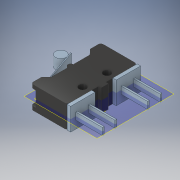
# Autodesk Inventor part: CH_01_0025_end_switch
Saved by Autodesk Inventor 2019 (Build 230136000, 136)
## iProperties
Created: 2022-03-07
Part Number: CH_01_0025_end_switch
Material: Generic
Document SubType Name: Modeling
Designer: Tomasz Krakowski
Density: 1 g/cm^3
Appearance: Default
Author: Tomasz Krakowski
Autodesk Inventor part; units mm, degrees
ref_plane "YZ Plane" through (0, 0, 0) normal (1, 0, 0) x (0, 1, 0)
ref_plane "XZ Plane" through (0, 0, 0) normal (0, 1, 0) x (-1, 0, 0)
ref_plane "XY Plane" through (0, 0, 0) normal (0, 0, 1) x (1, 0, 0)
sketch "Sketch1" plane through (0, 0, 0) normal (0, 1, 0) x (-1, 0, 0)
  line L0 (0, 0) -> (0, 1)
  line L1 (0, 1) -> (0.75, 1)
  line L2 (0.75, 1) -> (0.75, 9.27)
  line L3 (1.5, 10.02) -> (10.4, 10.02)
  line L4 (11.15, 9.27) -> (11.15, 7.02)
  line L5 (11.15, 7.02) -> (9.75, 5.5)
  line L6 (9.75, 5.5) -> (9.75, 0.75)
  arc A0 (10.5, 0) -> (9.75, 0.75) centre (9.75, 0) ccw
  line L7 (9.75, 0) -> (9.75, 0.75) construction
  circle A1 centre (2.85, 3.5) radius 1.05
  line L8 (9.75, 0) -> (9.25, 0) construction
  line L9 (0, 0) -> (9.25, 0) construction
  line L10 (9.75, 7.7) -> (9.75, 5.5) construction
  arc A2 (11.15, 9.27) -> (10.4, 10.02) centre (10.4, 9.27) ccw
  arc A3 (1.5, 10.02) -> (0.75, 9.27) centre (1.5, 9.27) ccw
  line L11 (9.75, 0) -> (10.5, 0) construction
  line L12 (0, 0) -> (0, -1)
  line L13 (0, -1) -> (0.75, -1)
  line L14 (0.75, -1) -> (0.75, -9.27)
  line L15 (1.5, -10.02) -> (10.4, -10.02)
  line L16 (11.15, -9.27) -> (11.15, -7.02)
  line L17 (11.15, -7.02) -> (9.75, -5.5)
  line L18 (9.75, -5.5) -> (9.75, -0.75)
  arc A4 (9.75, -0.75) -> (10.5, 0) centre (9.75, 0) ccw
  line L19 (9.75, 0) -> (9.75, -0.75) construction
  circle A5 centre (2.85, -3.5) radius 1.05
  line L20 (9.75, -7.7) -> (9.75, -5.5) construction
  arc A6 (10.4, -10.02) -> (11.15, -9.27) centre (10.4, -9.27) ccw
  arc A7 (0.75, -9.27) -> (1.5, -10.02) centre (1.5, -9.27) ccw
  point P0 (11.15, 10.02)
  point P1 (11.15, -10.02)
  dimension "d0" = 0.75
  dimension "d1" = 2.1
  dimension "d2" = 3.5
  dimension "d3" = 10.02
  dimension "d4" = 3
  dimension "d5" = 0.75
  dimension "d6" = 2.1
  dimension "d7" = 1
  dimension "d8" = 6.9
  dimension "d9" = 8.3
  dimension "d10" = 4.2
  dimension "d11" = 5.5
  dimension "d12" = 0.75
  constraints: 42 end point, 14 symmetric about line, 12 point on circle, 8 centre point, 4 perpendicular, 4 point on line, 4 tangent, 3 collinear, 2 horizontal, 1 equal radius, 1 parallel, 1 vertical, 4 other
  measures "d0" distance of L6.end L7.start
  measures "d1" distance from line of L2 A1.centre
  measures "d2" vertical distance of L0.start A1.centre
  measures "d3" distance from line of L0.start L3
  measures "d4" distance of point (11.15, 10.02) L4.end
  measures "d5" distance of L0.end L1.end
  measures "d6" diameter of A1
  measures "d7" distance between parallel lines of L9 L1
  measures "d8" distance from line of A1.centre L6
  measures "d9" distance from line of L4 A1.centre
  measures "d10" vertical distance of A1.centre L10.start
  measures "d11" distance from line of L8 L5.end
  measures "d12" radius of A2
extrude "Extrusion1" add sketch "Sketch1" along normal blind 6.4
sketch "Sketch2" plane through (-0.75, 0, 9.27) normal (1, 0, 0) x (0, 0, -1)
  line L0 (-0.75, 0) -> (0, 0) projected
  line L1 (8.52, 6.4) -> (3.77, 6.4) construction
  line L2 (-0.75, 0) -> (6.25, 0)
  line L3 (6.25, 0) -> (6.25, 6.4)
  line L4 (6.25, 6.4) -> (-0.75, 6.4)
  line L5 (-0.75, 6.4) -> (-0.75, 0)
  line L6 (8.27, 6.4) -> (10.27, 6.4) construction
  line L7 (9.27, 6.4) -> (9.27, 0) construction
  line L8 (19.29, 0) -> (18.54, 0)
  line L9 (19.29, 0) -> (12.29, 0)
  line L10 (12.29, 0) -> (12.29, 6.4)
  line L11 (12.29, 6.4) -> (19.29, 6.4)
  line L12 (19.29, 6.4) -> (19.29, 0)
  point P0 (14.77, 6.4)
  dimension "d15" = 7
  constraints: 20 end point, 6 symmetric about line, 2 parallel, 1 horizontal, 1 midpoint, 1 perpendicular, 1 point on line, 1 vertical
  measures "d15" distance between parallel lines of L5 L3
extrude "Extrusion2" add sketch "Sketch2" along normal blind 1 separate body
sketch "Sketch3" plane through (0.25, 0, 9.27) normal (1, 0, 0) x (0, 0, -1)
  line L0 (0.75, 2.2) -> (1.25, 2.2)
  line L1 (1.25, 2.2) -> (1.25, 4.2)
  line L2 (1.25, 4.2) -> (0.75, 4.2)
  line L3 (0.75, 4.2) -> (0.75, 2.2)
  line L4 (0.75, 2.2) -> (1.25, 4.2) construction
  line L5 (1.25, 2.2) -> (0.75, 4.2) construction
  line L6 (4.35, 2.2) -> (4.85, 2.2)
  line L7 (4.85, 2.2) -> (4.85, 4.2)
  line L8 (4.85, 4.2) -> (4.35, 4.2)
  line L9 (4.35, 4.2) -> (4.35, 2.2)
  line L10 (4.35, 2.2) -> (4.85, 4.2) construction
  line L11 (4.85, 2.2) -> (4.35, 4.2) construction
  line L12 (1, 3.2) -> (4.6, 3.2) construction
  line L13 (-0.75, 0) -> (-0.75, 6.4) construction
  line L14 (-0.75, 3.2) -> (1, 3.2) construction
  point P0 (9.27, 0)
  dimension "d18" = 0.5
  dimension "d19" = 2
  dimension "d21" = 3.6
  dimension "d22" = 1.75
  constraints: 28 end point, 5 midpoint, 4 parallel, 3 collinear, 3 horizontal, 2 perpendicular
  measures "d18" distance of L1.end L2.end
  measures "d19" distance between parallel lines of L0 L2
  measures "d21" distance of L12.end L12.start
  measures "d22" distance of L14.start L12.start
extrude "Extrusion3" add sketch "Sketch3" along normal blind 7.6 bodies 2
mirror "Mirror1" about plane through (0, 0, 0) normal (0, 0, 1) of "Extrusion3" bodies 2
sketch "Sketch4" plane through (-1.5, 0, -10.02) normal (0, 0, -1) x (-1, 0, 0)
  line L0 (9.65, 0) -> (9.65, 6.4) construction
  line L1 (9.65, 5.4) -> (8.25, 5.4)
  line L2 (8.25, 5.4) -> (8.25, 1)
  line L3 (8.25, 1) -> (9.65, 1)
  line L4 (9.65, 1) -> (9.65, 5.4)
  line L5 (8.25, 0) -> (8.25, 6.4) construction
  point P0 (-1.5, 0)
  dimension "d25" = 1
  dimension "d26" = 1
  constraints: 8 end point, 2 parallel, 1 collinear, 1 horizontal, 1 perpendicular, 1 point on line
  measures "d25" distance from line of L0.end L1
  measures "d26" distance from line of L0.start L3
extrude "Extrusion4" cut sketch "Sketch4" against normal through all bodies 1
sketch "Sketch5" plane through (0, 0, 0) normal (0, 1, 0) x (-1, 0, 0)
  point P0 (0, 0)
ref_plane "Work Plane1" through (-9.75, 3.2, 10.02) normal (0, -1, 0) x (1, 0, 0)
sketch "Sketch6" plane through (-9.75, 3.2, 10.02) normal (0, -1, 0) x (1, 0, 0)
  line L0 (-0.4, -1.6) -> (-5.0173, -14.9226)
  circle A0 centre (-5.9959, -13.1657) radius 1.5
  line L1 (0, -4.52) -> (0, 0) construction
  line L2 (-0.4, -1.6) -> (-0.1647, -1.6816)
  line L3 (-0.1647, -1.6816) -> (-4.7819, -15.0041)
  line L4 (-4.7819, -15.0041) -> (-5.0173, -14.9226)
  point P0 (9.75, -10.02)
  dimension "d29" = 14.1
  dimension "d30" = 0.4
  dimension "d31" = 1.6
  dimension "d32" = 3
  constraints: 8 end point, 2 perpendicular, 1 centre point, 1 parallel, 1 tangent
  measures "d29" distance of L0.end L0.start
  measures "d30" distance from line of L1 L0.start
  measures "d31" vertical distance of L1.end L0.start
  measures "d32" diameter of A0
extrude "Extrusion5" add sketch "Sketch6" along normal mid plane 3 separate body
equation "\"d26\" = d25"
body "Solid1"
body "Solid2"
body "Solid3"
